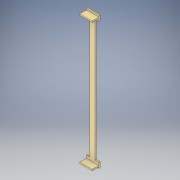
# Autodesk Inventor part: Cover v1x
Saved by Autodesk Inventor 2019 (Build 230136000, 136)
## iProperties
Created: 2021-07-14
Part Number: Cover v1x
Material: Generic
Document SubType Name: Modeling
Designer: Lix
Density: 1 g/cm^3
Appearance: Beige
Author: Lix
Autodesk Inventor part; units mm, degrees
ref_plane "YZ Plane" through (0, 0, 0) normal (1, 0, 0) x (0, 1, 0)
ref_plane "XZ Plane" through (0, 0, 0) normal (0, 1, 0) x (-1, 0, 0)
ref_plane "XY Plane" through (0, 0, 0) normal (0, 0, 1) x (1, 0, 0)
sketch "Sketch1" plane through (0, 0, 0) normal (0, 0, 1) x (1, 0, 0)
  line L0 (57.735, -100) -> (-57.735, -100)
  line L1 (-57.735, -100) -> (-115.4701, 0)
  line L2 (-115.4701, 0) -> (-57.735, 100)
  line L3 (-57.735, 100) -> (57.735, 100)
  line L4 (57.735, 100) -> (115.4701, 0)
  line L5 (115.4701, 0) -> (57.735, -100)
  point P0 (0, 0)
  point P1 (0, 0)
  dimension "d0" = 200
  constraints: 12 end point, 1 coincident, 1 horizontal, 13 other
  measures "d0" distance between parallel lines of L4 L1
extrude "Extrusion1" add sketch "Sketch1" along normal blind 2
sketch "Sketch5" plane through (0, 0, 2) normal (0, 0, 1) x (1, 0, 0)
  line L0 (-57.735, -100) -> (57.735, -100) projected
  line L1 (57.735, -100) -> (115.4701, 0) projected
  line L2 (115.4701, 0) -> (57.735, 100) projected
  line L3 (57.735, 100) -> (-57.735, 100) projected
  line L4 (-57.735, 100) -> (-115.4701, 0) projected
  line L5 (-115.4701, 0) -> (-57.735, -100) projected
  line L6 (-113.1607, 0) -> (-56.5803, 98)
  line L7 (-56.5803, 98) -> (56.5803, 98)
  line L8 (56.5803, 98) -> (113.1607, 0)
  line L9 (113.1607, 0) -> (56.5803, -98)
  line L10 (56.5803, -98) -> (-56.5803, -98)
  line L11 (-56.5803, -98) -> (-113.1607, 0)
  line L12 (-110.8513, 0) -> (-55.4256, 96)
  line L13 (-55.4256, 96) -> (55.4256, 96)
  line L14 (55.4256, 96) -> (110.8513, 0)
  line L15 (110.8513, 0) -> (55.4256, -96)
  line L16 (55.4256, -96) -> (-55.4256, -96)
  line L17 (-55.4256, -96) -> (-110.8513, 0)
  point P0 (0, 0)
  dimension "d15" = 2
  dimension "d16" = 2
  constraints: 24 end point, 10 other
  measures "d15" distance between parallel lines of L4 L6
  measures "d16" distance between parallel lines of L11 L17
extrude "Extrusion5" add sketch "Sketch5" along normal blind 10 contours L6 L7 L8 L9 L10 L11
sketch "Sketch7" plane through (0, 0, 2) normal (0, 0, 1) x (1, 0, 0)
  line L0 (55.4256, 96) -> (-55.4256, 96) projected
  line L1 (-55.4256, 96) -> (-110.8513, 0) projected
  line L2 (-110.8513, 0) -> (-55.4256, -96) projected
  line L3 (-55.4256, -96) -> (55.4256, -96) projected
  line L4 (55.4256, -96) -> (110.8513, 0) projected
  line L5 (110.8513, 0) -> (55.4256, 96) projected
  line L6 (-53.1162, -92) -> (-106.2324, 0)
  line L7 (-106.2324, 0) -> (-53.1162, 92)
  line L8 (-53.1162, 92) -> (53.1162, 92)
  line L9 (53.1162, 92) -> (106.2324, 0)
  line L10 (106.2324, 0) -> (53.1162, -92)
  line L11 (53.1162, -92) -> (-53.1162, -92)
  point P0 (0, 0)
  dimension "d19" = 4
  constraints: 12 end point, 5 other
  measures "d19" distance between parallel lines of L2 L6
extrude "Extrusion6" cut sketch "Sketch7" against normal blind 7 contours L6 L7 L8 L9 L10 L11
fillet "Fillet1" radius 10 6 edges at (57.735, 100, 1) (115.4701, 0, 1) (57.735, -100, 1) (-57.735, -100, 1) (-115.4701, 0, 1) (-57.735, 100, 1)
fillet "Fillet1" radius 4 12 edges at (56.5803, -98, 7) (-55.4256, -96, 7) (-113.1607, 0, 7) (-56.5803, 98, 7) (56.5803, 98, 7) (113.1607, 0, 7) (55.4256, -96, 7) (110.8513, 0, 7) (-55.4256, 96, 7) (55.4256, 96, 7) (-56.5803, -98, 7) (-110.8513, 0, 7)
fillet "Fillet2" radius 10 6 edges at (53.1162, -92, 1) (106.2324, 0, 1) (53.1162, 92, 1) (-53.1162, 92, 1) (-106.2324, 0, 1) (-53.1162, -92, 1)
sketch "Sketch8" plane through (0, 0, 2) normal (0, 0, 1) x (1, 0, 0)
  arc A0 (-109.6966, 2) -> (-109.6966, -2) centre (-106.2324, 0) ccw projected
  line L0 (-109.6966, -2) -> (-56.5803, -94) projected
  arc A1 (-56.5803, -94) -> (-53.1162, -96) centre (-53.1162, -92) ccw projected
  line L1 (-53.1162, -96) -> (53.1162, -96) projected
  arc A2 (53.1162, -96) -> (56.5803, -94) centre (53.1162, -92) ccw projected
  line L2 (56.5803, -94) -> (109.6966, -2) projected
  arc A3 (109.6966, -2) -> (109.6966, 2) centre (106.2324, 0) ccw projected
  line L3 (109.6966, 2) -> (56.5803, 94) projected
  arc A4 (56.5803, 94) -> (53.1162, 96) centre (53.1162, 92) ccw projected
  line L4 (53.1162, 96) -> (-53.1162, 96) projected
  arc A5 (-53.1162, 96) -> (-56.5803, 94) centre (-53.1162, 92) ccw projected
  line L5 (-56.5803, 94) -> (-109.6966, 2) projected
  line L6 (47.3427, -92) -> (-47.3427, -92) projected
  arc A6 (-56.003, -87) -> (-47.3427, -92) centre (-47.3427, -82) ccw projected
  line L7 (-56.003, -87) -> (-103.3457, -5) projected
  arc A7 (-103.3457, 5) -> (-103.3457, -5) centre (-94.6854, 0) ccw projected
  line L8 (-103.3457, 5) -> (-56.003, 87) projected
  arc A8 (-47.3427, 92) -> (-56.003, 87) centre (-47.3427, 82) ccw projected
  line L9 (-47.3427, 92) -> (47.3427, 92) projected
  arc A9 (56.003, 87) -> (47.3427, 92) centre (47.3427, 82) ccw projected
  line L10 (56.003, 87) -> (103.3457, 5) projected
  arc A10 (103.3457, -5) -> (103.3457, 5) centre (94.6854, 0) ccw projected
  line L11 (103.3457, -5) -> (56.003, -87) projected
  arc A11 (47.3427, -92) -> (56.003, -87) centre (47.3427, -82) ccw projected
  line L12 (-47.3427, -92) -> (47.3427, -92) projected
  line L13 (-4, -92) -> (4, -92)
  line L14 (4, -92) -> (4, 92)
  line L15 (4, 92) -> (-4, 92)
  line L16 (-4, 92) -> (-4, -92)
  point P0 (0, 0)
  dimension "d25" = 4
  dimension "d26" = 4
  constraints: 8 end point, 2 parallel, 2 point on line, 1 horizontal, 1 perpendicular
  measures "d25" distance from line of L16 point (0, 0)
  measures "d26" distance from line of L14 point (0, 0)
extrude "Extrusion7" add sketch "Sketch8" against normal up to surface (2 mm away) contours L6 L16 L9 L14
sketch "Sketch9" plane through (0, 0, 0) normal (0, 0, -1) x (-1, 0, 0)
  line L0 (199.1804, 180.8963) -> (8.9476, 180.8963)
  line L1 (8.9476, 180.8963) -> (8.9476, -184.7865)
  line L2 (8.9476, -184.7865) -> (199.1804, -184.7865)
  line L3 (199.1804, -184.7865) -> (199.1804, 180.8963)
  line L4 (-233.8036, -220.5767) -> (-9.7256, -220.5767)
  line L5 (-9.7256, -220.5767) -> (-9.7256, 196.8463)
  line L6 (-9.7256, 196.8463) -> (-233.8036, 196.8463)
  line L7 (-233.8036, 196.8463) -> (-233.8036, -220.5767)
  point P0 (0, 0)
  constraints: 16 end point, 4 parallel, 2 horizontal, 2 perpendicular
extrude "Extrusion8" cut sketch "Sketch9" against normal blind 20
equation "\"d26\" = d25"
body "Solid1"
